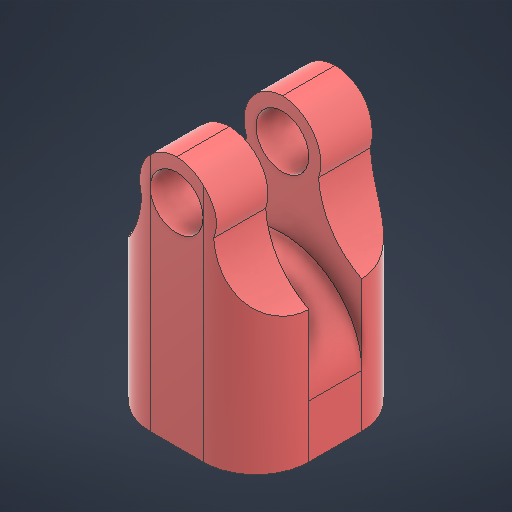
# Autodesk Inventor part: Connector_hollow
Saved by Autodesk Inventor 2027 (Build 310192060, 192F)
## iProperties
Created: 2026-08-01
Part Number: Connector_hollow
Material: Ogólny
Document SubType Name: Modeling
Designer: User
Density: 1 g/cm^3
Appearance: Domyślna
Author: User
Autodesk Inventor part; units mm, degrees
ref_plane "YZ Plane" through (0, 0, 0) normal (1, 0, 0) x (0, 1, 0)
ref_plane "XZ Plane" through (0, 0, 0) normal (0, 1, 0) x (-1, 0, 0)
sketch "Szkic3" plane through (0, 0, 0) normal (0, 1, 0) x (-1, 0, 0)
  circle A0 centre (0, 0) radius 5
  line L0 (-6, -6) -> (6, -6)
  line L1 (6, -6) -> (6, 6)
  line L2 (6, 6) -> (-6, 6)
  line L3 (-6, 6) -> (-6, -6)
  line L4 (-6, -6) -> (6, 6) construction
  line L5 (6, -6) -> (-6, 6) construction
  dimension "d12" = 10
  dimension "d15" = 12
  dimension "d16" = 12
  constraints: 12 end point, 2 midpoint, 2 parallel, 1 centre point, 1 coincident, 1 horizontal, 1 perpendicular
  measures "d12" diameter of A0
  measures "d15" distance of L2.end L1.end
  measures "d16" distance of L1.end L0.end
extrude "Wyciągnięcie proste3" add sketch "Szkic3" along normal mid plane 10
extrude "Wyciągnięcie proste4" add sketch "Szkic3" along normal blind 5 contours A0
ref_plane "Płaszczyzna konstrukcyjna2" through (-6, 5, 0) normal (0, 0, 1) x (1, 0, 0)
sketch "Szkic7" plane through (-6, 5, 0) normal (0, 0, 1) x (1, 0, 0)
  line L0 (0, 0) -> (12, 0) projected
  line L1 (0, 0) -> (12, 0)
  line L2 (6, 0) -> (6, 6)
  line L3 (6, 0) -> (12, 0) construction
  circle A0 centre (6, 6) radius 2
  line L4 (4.2679, 5) -> (3.2679, 5)
  line L5 (6, 8) -> (6, 9)
  line L6 (7.7321, 5) -> (8.7321, 5)
  arc A1 (0, 0) -> (3.2679, 5) centre (-2.722, 5.347) ccw
  arc A2 (6, 9) -> (3.2679, 5) centre (6.0958, 6.0015) ccw
  arc A3 (8.7321, 5) -> (6, 9) centre (5.9042, 6.0015) ccw
  arc A4 (8.7321, 5) -> (12, 0) centre (14.722, 5.347) ccw
  point P0 (6, -5)
  dimension "d42" = 6
  dimension "d43" = 90
  dimension "d44" = 4
  dimension "d45" = 1
  dimension "d46" = 1
  dimension "d47" = 1
  dimension "d48" = 5
  dimension "d49" = 5
  dimension "d50" = 0
  dimension "d51" = 6
  dimension "d52" = 3
  dimension "d53" = 3
  dimension "d54" = 6
  constraints: 12 end point, 11 point on circle, 5 centre point, 3 horizontal, 2 vertical, 1 coincident, 1 collinear, 1 midpoint, 1 perpendicular
  measures "d42" distance of L2.start L2.end
  measures "d43" angle of L3 L2
  measures "d44" diameter of A0
  measures "d45" distance of L4.start L4.end
  measures "d46" distance of L5.start L5.end
  measures "d47" distance of L6.start L6.end
  measures "d48" distance between parallel lines of L6 L0
  measures "d49" distance between parallel lines of L4 L0
  measures "d50" distance between parallel lines of L5 L2
  measures "d51" radius of A1
  measures "d52" radius of A2
  measures "d53" radius of A3
  measures "d54" radius of A4
extrude "Wyciągnięcie proste7" add sketch "Szkic7" along normal mid plane 12 contours A1 L4 A0 L2 L0 | L2 A0 L6 A4 L0 | A2 L5 A0 L4 | A3 L6 A0 L5
sketch "Szkic8" plane through (-6, 5, 0) normal (0, 0, 1) x (1, 0, 0)
  arc A0 (8.7321, 5) -> (12, 0) centre (14.722, 5.347) ccw projected
  line L0 (0, 12) -> (12, 12)
  line L1 (12, 12) -> (12, 0)
  line L2 (12, 0) -> (0, 0)
  line L3 (0, 0) -> (0, 12)
  circle A1 centre (6, 6) radius 2 projected
  line L4 (0, 12) -> (12, 0) construction
  line L5 (12, 12) -> (0, 0) construction
  point P0 (6, -5)
  constraints: 12 end point, 2 midpoint, 2 parallel, 1 horizontal, 1 perpendicular
extrude "Wyciągnięcie proste8" cut sketch "Szkic8" along normal mid plane 4
fillet "Zaokrąglenie5" radius 6 2 edges at (6, 5, 0) (-6, 5, 0)
fillet "Zaokrąglenie6" radius 4 4 edges at (6, 0, 6) (6, 0, -6) (-6, 0, -6) (-6, 0, 6)
